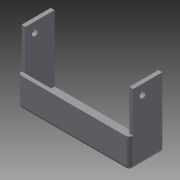
# Autodesk Inventor part: Back_Shield
Saved by Autodesk Inventor 2014 (Build 180170000, 170)
## iProperties
Created: 2014-05-02
Part Number: Back_Shield
Material: Generic
Document SubType Name: Modeling
Designer: Alex
Density: 1 g/cm^3
Appearance: Default
Author: Alex
Autodesk Inventor part; units mm, degrees
ref_plane "YZ Plane" through (0, 0, 0) normal (1, 0, 0) x (0, 1, 0)
ref_plane "XZ Plane" through (0, 0, 0) normal (0, 1, 0) x (-1, 0, 0)
ref_plane "XY Plane" through (0, 0, 0) normal (0, 0, 1) x (1, 0, 0)
sketch "Sketch1" plane through (0, 0, 0) normal (0, 0, 1) x (1, 0, 0)
  line L0 (0, 0) -> (68.58, 0)
  line L1 (68.58, 0) -> (68.58, 17.018)
  line L2 (68.58, 17.018) -> (0, 17.018)
  line L3 (0, 17.018) -> (0, 0)
  dimension "d0" = 17.018
  dimension "d1" = 68.58
  constraints: 8 end point, 2 parallel, 1 horizontal, 1 perpendicular
  measures "d0" distance of L2.end L0.start
  measures "d1" distance of L0.start L0.end
extrude "Extrusion1" add sketch "Sketch1" along normal blind 2.54
sketch "Sketch2" plane through (0, 0, 2.54) normal (0, 0, 1) x (1, 0, 0)
  line L0 (0, 0) -> (68.58, 0) projected
  line L1 (68.58, 0) -> (68.58, 17.018) projected
  line L2 (68.58, 17.018) -> (0, 17.018) projected
  line L3 (0, 17.018) -> (0, 0) projected
  line L4 (-2.54, 17.018) -> (71.12, 17.018)
  line L5 (71.12, 17.018) -> (71.12, -2.54)
  line L6 (71.12, -2.54) -> (-2.54, -2.54)
  line L7 (-2.54, -2.54) -> (-2.54, 17.018)
  dimension "d4" = 0
  dimension "d5" = 2.54
  dimension "d6" = 2.54
  dimension "d7" = 2.54
  constraints: 8 end point, 2 parallel, 1 horizontal, 1 perpendicular
  measures "d4" distance between parallel lines of L2 L4
  measures "d5" distance between parallel lines of L3 L7
  measures "d6" distance between parallel lines of L5 L1
  measures "d7" distance between parallel lines of L6 L0
extrude "Extrusion2" add sketch "Sketch2" against normal blind 21.844 contours L0 L1 L4 L5 L6 L7 L3
fillet "Fillet1" radius 2.54 5 edges at (71.12, -2.54, -8.382) (-2.54, -2.54, -8.382) (34.29, -2.54, 2.54) (71.12, 7.239, 2.54) (-2.54, 7.239, 2.54)
sketch "Sketch3" plane through (0, 17.018, 0) normal (0, 1, 0) x (1, 0, 0)
  arc A0 (68.58, -2.54) -> (71.12, 0) centre (68.58, 0) ccw projected
  arc A1 (-2.54, 0) -> (0, -2.54) centre (0, 0) ccw projected
  line L0 (-2.54, 19.304) -> (0, 19.304)
  line L1 (0, 19.304) -> (0, 0)
  line L2 (0, 0) -> (-2.54, 0)
  line L3 (-2.54, 0) -> (-2.54, 19.304)
  line L4 (68.58, 0) -> (71.12, 0)
  line L5 (71.12, 0) -> (71.12, 19.304)
  line L6 (71.12, 19.304) -> (68.58, 19.304)
  line L7 (68.58, 19.304) -> (68.58, 0)
  constraints: 16 end point, 4 parallel, 2 horizontal, 2 perpendicular
extrude "Extrusion3" add sketch "Sketch3" along normal blind 26.67
hole "Hole1" at (71.12, 37.338, -6.35) direction (-1, 0, 0) diameter 4.1656 end through all
equation "\"d6\" = d5"
equation "\"d7\" = d6"
body "Solid1"
